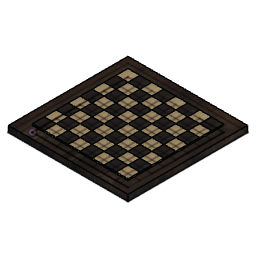
Chess Board (Autodesk Fusion 360 design; units mm, degrees)
Autodesk Fusion 360 part; units mm, degrees
sketch "Chess Board" plane through (0, 0, 0) normal (0, 0, 1) x (1, 0, 0)
  line L0 (0, 0) -> (320, 0)
  line L1 (320, 0) -> (320, 320)
  line L2 (320, 320) -> (0, 320)
  line L3 (0, 320) -> (0, 0)
  line L4 (0, 160) -> (320, 160)
  line L5 (160, 0) -> (160, 320)
  line L6 (0, 0) -> (160, 0)
  line L7 (80, 0) -> (80, 320)
  line L8 (160, 0) -> (320, 0)
  line L9 (240, 0) -> (240, 320)
  line L10 (320, 320) -> (320, 160)
  line L11 (320, 240) -> (0, 240)
  line L12 (0, 160) -> (0, 0)
  line L13 (0, 80) -> (320, 80)
  line L14 (0, 0) -> (80, 0)
  line L15 (40, 0) -> (40, 320)
  line L16 (160, 0) -> (80, 0)
  line L17 (120, 0) -> (120, 320)
  line L18 (160, 0) -> (240, 0)
  line L19 (200, 0) -> (200, 320)
  line L20 (240, 320) -> (320, 320)
  line L21 (240, 0) -> (320, 0)
  line L22 (280, 0) -> (280, 320)
  line L23 (320, 160) -> (320, 80)
  line L24 (0, 160) -> (0, 80)
  line L25 (0, 120) -> (320, 120)
  line L26 (0, 240) -> (0, 160)
  line L27 (320, 160) -> (320, 240)
  line L28 (0, 200) -> (320, 200)
  line L29 (0, 80) -> (0, 0)
  line L30 (0, 40) -> (320, 40)
  line L31 (0, 240) -> (0, 320)
  line L32 (320, 240) -> (320, 320)
  line L33 (0, 280) -> (320, 280)
  line L34 (360, -40) -> (360, 360)
  line L35 (360, 360) -> (-40, 360)
  line L36 (-40, 360) -> (-40, -40)
  line L37 (-40, -40) -> (360, -40)
  dimension "d1" = 320
  dimension "d2" = 320
  dimension "d3" = 40
  constraint horizontal L0
  constraint vertical L1
  constraint horizontal L2
  constraint vertical L3
  constraint coincident L0.start L3.end
  constraint midpoint L3 L4.start
  constraint midpoint L1 L4.end
  constraint midpoint L0 L5.start
  constraint midpoint L2 L5.end
  constraint midpoint L6 L7.start
  constraint coincident L2 L7.end
  constraint perpendicular L2 L7
  constraint midpoint L8 L9.start
  constraint coincident L2 L9.end
  constraint perpendicular L2 L9
  constraint midpoint L10 L11.start
  constraint coincident L3 L11.end
  constraint perpendicular L3 L11
  constraint midpoint L12 L13.start
  constraint coincident L1 L13.end
  constraint perpendicular L1 L13
  constraint midpoint L14 L15.start
  constraint coincident L2 L15.end
  constraint perpendicular L2 L15
  constraint midpoint L16 L17.start
  constraint coincident L2 L17.end
  constraint perpendicular L2 L17
  constraint midpoint L18 L19.start
  constraint coincident L2 L19.end
  constraint perpendicular L2 L19
  constraint midpoint L21 L22.start
  constraint midpoint L20 L22.end
  constraint midpoint L24 L25.start
  constraint midpoint L23 L25.end
  constraint midpoint L26 L28.start
  constraint midpoint L27 L28.end
  constraint midpoint L29 L30.start
  constraint coincident L1 L30.end
  constraint perpendicular L1 L30
  constraint midpoint L31 L33.start
  constraint midpoint L32 L33.end
  measures "d1" distance of L0.start L0.end
  measures "d2" distance of L0.start L2.end
extrude "Extrude1" add sketch "Chess Board" along normal blind 20 makes body 1
extrude "Extrude2" add sketch "Chess Board" along normal blind 25 separate body contours L0 L3 L6 L12 L14 L15 L29 L30 | L0 L6 L7 L16 L17 L30 | L7 L13 L15 L30 | L3 L12 L13 L15 L24 L25 | L0 L5 L8 L18 L19 L30 | L5 L13 L17 L30 | L7 L13 L17 L25 | L4 L7 L15 L25 | L3 L4 L15 L26 L28 | L0 L8 L9 L21 L22 L30 | L9 L13 L19 L30 | L5 L13 L19 L25 | L4 L5 L17 L25 | L4 L7 L17 L28 | L7 L11 L15 L28 | L3 L11 L15 L31 L33 | L1 L13 L22 L30 | L9 L13 L22 L25 | L4 L9 L19 L25 | L4 L5 L19 L28 | L5 L11 L17 L28 | L7 L11 L17 L33 | L2 L7 L15 L33 | L1 L4 L22 L23 L25 | L4 L9 L22 L28 | L9 L11 L19 L28 | L5 L11 L19 L33 | L2 L5 L17 L33 | L1 L10 L11 L22 L27 L28 | L9 L11 L22 L33 | L2 L9 L19 L33 makes body 2 at (13.3333, 26.6667, 0)
extrude "Extrude3" add sketch "Chess Board" along normal blind 25 separate body contours L0 L6 L7 L14 L15 L30 | L3 L12 L13 L15 L29 L30 | L0 L5 L6 L16 L17 L30 | L7 L13 L17 L30 | L7 L13 L15 L25 | L3 L4 L12 L15 L24 L25 | L0 L8 L9 L18 L19 L30 | L5 L13 L19 L30 | L5 L13 L17 L25 | L4 L7 L17 L25 | L4 L7 L15 L28 | L3 L11 L15 L26 L28 | L0 L1 L8 L21 L22 L30 | L9 L13 L22 L30 | L9 L13 L19 L25 | L4 L5 L19 L25 | L4 L5 L17 L28 | L7 L11 L17 L28 | L7 L11 L15 L33 | L2 L3 L15 L31 L33 | L1 L13 L22 L23 L25 | L4 L9 L22 L25 | L4 L9 L19 L28 | L5 L11 L19 L28 | L5 L11 L17 L33 | L2 L7 L17 L33 | L1 L4 L10 L22 L27 L28 | L9 L11 L22 L28 | L9 L11 L19 L33 | L2 L5 L19 L33 | L1 L10 L11 L22 L32 L33 | L2 L9 L20 L22 L33 makes body 3 at (53.3333, 26.6667, 0)
extrude "Extrude4" add sketch "Chess Board" along normal blind 24 separate body contours L1 L2 L10 L20 L22 L32 L33 makes body 4
combine "Combine1" operation add target body 4 tool bodies 2
named bodies: "Border", "White", "Black"
